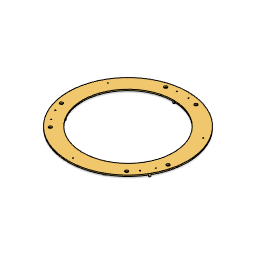
Hexapod Assembly (v6~recovered) (Autodesk Fusion 360 archive; units mm, degrees)
design "Bottom Plate"
Autodesk Fusion 360 part; units mm, degrees
sketch "Sketch1" plane through (0, 0, 0) normal (0, 1, 0) x (1, 0, 0)
  circle A0 centre (0, 0) radius 250
  circle A1 centre (0, 0) radius 230 construction
  circle A2 centre (63.3966, 221.0902) radius 6.5
  line L0 (63.3966, 221.0902) -> (0, 0) construction
  line L1 (0, 0) -> (0, 284.6738) construction
  line L2 (0, 0) -> (360.2208, 0) construction
  circle A3 centre (-63.3966, 221.0902) radius 6.5
  circle A4 centre (-223.168, -55.642) radius 6.5
  circle A5 centre (-159.7714, -165.4482) radius 6.5
  circle A6 centre (159.7714, -165.4482) radius 6.5
  circle A7 centre (223.168, -55.642) radius 6.5
  dimension "d13" = 500
  dimension "d14" = 460
  dimension "d15" = 13
  dimension "d60" = 16
  dimension "d62" = 360
  constraint coincident A0.centre A1.centre
  constraint concentric A0 A1
  constraint coincident A1 A2.centre
  constraint coincident A2.centre L0.start
  constraint vertical L1
  constraint perpendicular L1 L2
  constraint symmetric A2 L1 A3
  measures "d13" diameter of A0
  measures "d14" diameter of A1
  measures "d15" diameter of A2
  measures "d60" angle of L0 L1
extrude "Extrude8" add sketch "Sketch1" along normal blind 5
extrude "Extrude2" add sketch "Sketch1" along normal blind 5 contours A0 | A3 | A4 | A5 | A6 | A7
sketch "Sketch2" plane through (0, 0, 0) normal (0, -1, 0) x (1, 0, 0)
  circle A0 centre (63.3966, -221.0902) radius 6.5
  circle A1 centre (0, 0) radius 250
  circle A2 centre (0, 0) radius 230
  line L0 (0, 0) -> (-199.1858, -115) construction
  line L1 (0, 0) -> (0, -250) construction
  circle A3 centre (-199.1858, -115) radius 12.5
  circle A4 centre (199.1858, -115) radius 12.5
  circle A5 centre (0, 230) radius 12.5
  dimension "d21" = 460
  dimension "d22" = 60
  dimension "d23" = 25
  dimension "d25" = 360
  constraint coincident A1.centre A2.centre
  constraint coincident A2 L0.end
  constraint coincident A1 L1.end
  constraint vertical L1
  constraint coincident L0.end A3.centre
  measures "d21" diameter of A2
  measures "d22" angle of L0 L1
  measures "d23" diameter of A3
hole "Hole1" at (-199.1858, -7, -115) direction (0, 1, 0) diameter 4 depth 20 tip angle 180
pattern_circular "C-Pattern1" count 3 over 360 about axis through (0, 1.75, 0) along (0, 1, 0) of "Hole1"
sketch "Sketch3" plane through (0, 0, 0) normal (0, -1, 0) x (1, 0, 0)
  circle A0 centre (63.3966, -221.0902) radius 6.5
  circle A1 centre (0, 0) radius 250
  circle A2 centre (0, 0) radius 250
  circle A3 centre (0, 0) radius 12.5
  line L0 (-3, -12.1347) -> (-3, -249.982)
  line L1 (3, -12.1347) -> (3, -249.982)
  line L2 (12.0089, 3.4693) -> (217.9908, 122.3929)
  line L3 (9.0089, 8.6654) -> (214.9908, 127.5891)
  line L4 (-9.0089, 8.6654) -> (-214.9908, 127.5891)
  line L5 (-12.0089, 3.4693) -> (-217.9908, 122.3929)
  circle A4 centre (199.1858, -115) radius 2
  circle A5 centre (0, 230) radius 2
  circle A6 centre (-199.1858, -115) radius 2
  dimension "d34" = 500
  dimension "d42" = 25
  dimension "d45" = 6
  dimension "d48" = 360
  constraint concentric A1 A2
  constraint coincident A3 L0.start
  constraint coincident A1 L0.end
  constraint vertical L0
  constraint coincident A3 L1.start
  constraint coincident A1 L1.end
  constraint parallel L0 L1
  measures "d34" diameter of A2
  measures "d42" diameter of A3
  measures "d45" distance of L0 L1
extrude "Extrude5" add sketch "Sketch3" along normal blind 7 contours A1 A2 A3 L2 L3 | A1 A2 A3 L0 L1 | A3 | A1 A2 A3 L4 L5
fillet "Fillet1" radius 3 6 edges at (-9.0089, -3.5, 8.6654) (9.0089, -3.5, 8.6654) (-3, -3.5, -12.1347) (-12.0089, -3.5, 3.4693) (12.0089, -3.5, 3.4693) (3, -3.5, -12.1347)
sketch "Sketch4" plane through (0, 0, 0) normal (0, -1, 0) x (1, 0, 0)
  arc A0 (4.8387, -11.5255) -> (3, -14.2916) centre (6, -14.2916) ccw
  line L0 (3, -14.2916) -> (3, -249.982)
  arc A1 (3, -249.982) -> (217.9908, 122.3929) centre (0, 0) ccw
  line L1 (217.9908, 122.3929) -> (13.8769, 4.5477)
  arc A2 (13.8769, 4.5477) -> (12.4007, 1.5723) centre (15.3769, 1.9497) ccw
  arc A3 (4.8387, -11.5255) -> (12.4007, 1.5723) centre (0, 0) ccw
  circle A4 centre (63.3966, -221.0902) radius 6.5
  circle A5 centre (0, 0) radius 250 construction
  circle A6 centre (0, 0) radius 230 construction
  circle A7 centre (186.0739, 135.1906) radius 2
  line L2 (0, 0) -> (0, 80) construction
  line L3 (186.0739, 135.1906) -> (0, 0) construction
  line L4 (0, 0) -> (216.5064, 125) construction
  circle A8 centre (210.1155, 93.5494) radius 2
  circle A9 centre (-186.0739, 135.1906) radius 2
  circle A10 centre (-210.1155, 93.5494) radius 2
  circle A11 centre (-24.0415, -228.74) radius 2
  circle A12 centre (24.0415, -228.74) radius 2
  circle A13 centre (229.8599, -8.0269) radius 12.5
  line L5 (229.8599, -8.0269) -> (0, 0) construction
  line L6 (0, 0) -> (275.6577, -159.151) construction
  circle A14 centre (121.8814, -195.0511) radius 12.5
  circle A15 centre (-107.9785, 203.0779) radius 12.5
  circle A16 centre (107.9785, 203.0779) radius 12.5
  circle A17 centre (-121.8814, -195.0511) radius 12.5
  circle A18 centre (-229.8599, -8.0269) radius 12.5
  circle A19 centre (199.1858, -115) radius 2
  circle A20 centre (229.8599, -8.0269) radius 2
  circle A21 centre (121.8814, -195.0511) radius 2
  circle A22 centre (107.9785, 203.0779) radius 2
  circle A23 centre (-107.9785, 203.0779) radius 2
  circle A24 centre (-229.8599, -8.0269) radius 2
  circle A25 centre (-121.8814, -195.0511) radius 2
  dimension "d53" = 460
  dimension "d54" = 4
  dimension "d55" = 54
  dimension "d57" = 360
  dimension "d65" = 500
  dimension "d73" = 25
  dimension "d74" = 32
  dimension "d75" = 28
  dimension "d77" = 360
  dimension "d80" = 4
  dimension "d82" = 360
  constraint concentric A1 A5
  constraint concentric A5 A6
  constraint coincident A6 A7.centre
  constraint coincident A1.centre A3.centre
  constraint vertical L2
  constraint coincident A7.centre L3.start
  constraint coincident A5 L4.end
  constraint parallel L1 L4
  constraint symmetric A7 L4 A8
  constraint coincident A6 A13.centre
  constraint coincident A13.centre L5.start
  constraint symmetric A13 L6 A14
  constraint concentric A13 A20
  constraint symmetric L6 A20 A21
  measures "d53" diameter of A6
  measures "d54" diameter of A7
  measures "d55" angle of L2 L3
  measures "d65" diameter of A5
  measures "d73" diameter of A13
  measures "d74" angle of L1 L5
  measures "d75" angle of L5 L6
  measures "d80" diameter of A20
extrude "Extrude11" add sketch "Sketch4" along normal blind 7 contours A13 | A14 | A15 | A16 | A17 | A18
extrude "Extrude6" cut sketch "Sketch4" against normal blind 40 contours A7 | A8 | A9 | A10 | A11 | A12
extrude "Extrude9" cut sketch "Sketch1" along normal blind 35 contours A2 | A3 | A4 | A5 | A6 | A7
sketch "Sketch5" plane through (0, -7, 0) normal (0, -1, 0) x (1, 0, 0)
  line L0 (-3, -14.2916) -> (-3, -249.982)
  arc A0 (-3, -249.982) -> (3, -249.982) centre (0, 0) ccw
  line L1 (3, -249.982) -> (3, -14.2916)
  arc A1 (4.8387, -11.5255) -> (3, -14.2916) centre (6, -14.2916) ccw
  arc A2 (4.8387, -11.5255) -> (12.4007, 1.5723) centre (0, 0) ccw
  arc A3 (13.8769, 4.5477) -> (12.4007, 1.5723) centre (15.3769, 1.9497) ccw
  line L2 (13.8769, 4.5477) -> (217.9908, 122.3929)
  arc A4 (217.9908, 122.3929) -> (214.9908, 127.5891) centre (0, 0) ccw
  line L3 (214.9908, 127.5891) -> (10.8769, 9.7439)
  arc A5 (7.562, 9.9532) -> (10.8769, 9.7439) centre (9.3769, 12.342) ccw
  arc A6 (7.562, 9.9532) -> (-7.562, 9.9532) centre (0, 0) ccw
  arc A7 (-10.8769, 9.7439) -> (-7.562, 9.9532) centre (-9.3769, 12.342) ccw
  line L4 (-10.8769, 9.7439) -> (-214.9908, 127.5891)
  arc A8 (-214.9908, 127.5891) -> (-217.9908, 122.3929) centre (0, 0) ccw
  line L5 (-217.9908, 122.3929) -> (-13.8769, 4.5477)
  arc A9 (-12.4007, 1.5723) -> (-13.8769, 4.5477) centre (-15.3769, 1.9497) ccw
  arc A10 (-12.4007, 1.5723) -> (-4.8387, -11.5255) centre (0, 0) ccw
  arc A11 (-3, -14.2916) -> (-4.8387, -11.5255) centre (-6, -14.2916) ccw
  circle A12 centre (0, 0) radius 190
  dimension "d70" = 380
  constraint concentric A0 A12
  measures "d70" diameter of A12
extrude "Extrude10" cut sketch "Sketch5" against normal blind 50 contours L0 L1 A1 A2 A3 L2 L3 A5 A6 A7 L4 L5 A9 A10 A11 A12 | L0 L5 A9 A10 A11 A12 | L1 A1 A2 A3 L2 A12 | L3 A5 A6 A7 L4 A12
equation "hole_angle = 16 deg"
equation "hole_c_diameter = 460 mm"
equation "disk_diameter = 500 mm"
equation "hole_diameter = 13 mm"
equation "d13 = disk_diameter"
equation "d14 = hole_c_diameter"
equation "d15 = hole_diameter"
equation "d21 = hole_c_diameter"
equation "d60 = hole_angle"
equation "d70 = disk_diameter - 120 mm"

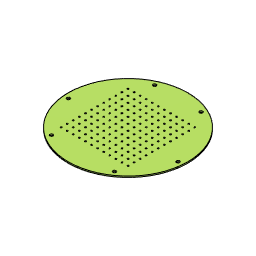
design "Top Plate"
Autodesk Fusion 360 part; units mm, degrees
sketch "Sketch2" plane through (0, 0, 0) normal (0, 1, 0) x (1, 0, 0)
  circle A0 centre (0, 0) radius 250
  circle A1 centre (0, 0) radius 230 construction
  line L0 (0, 0) -> (0, 300) construction
  circle A2 centre (97.2022, 208.4508) radius 6.5
  line L1 (97.2022, 208.4508) -> (0, 0) construction
  circle A3 centre (-97.2022, 208.4508) radius 6.5
  circle A4 centre (-229.1248, -20.0458) radius 6.5
  circle A5 centre (-131.9226, -188.405) radius 6.5
  circle A6 centre (131.9226, -188.405) radius 6.5
  circle A7 centre (229.1248, -20.0458) radius 6.5
  dimension "d52" = 500
  dimension "d53" = 460
  dimension "d54" = 13
  dimension "d55" = 25
  dimension "d57" = 360
  constraint coincident A0.centre A1.centre
  constraint vertical L0
  constraint coincident A1 A2.centre
  constraint coincident A2.centre L1.start
  constraint symmetric L0 A2 A3
  measures "d52" diameter of A0
  measures "d53" diameter of A1
  measures "d54" diameter of A2
  measures "d55" angle of L0 L1
extrude "Extrude4" add sketch "Sketch2" along normal blind 5
sketch "Sketch3" plane through (0, 5, 0) normal (0, 1, 0) x (-1, 0, 0)
  circle A0 centre (-97.2022, -208.4508) radius 6.5
  circle A1 centre (229.1248, 20.0458) radius 6.5
  circle A2 centre (97.2022, -208.4508) radius 6.5
  circle A3 centre (131.9226, 188.405) radius 6.5
  circle A4 centre (-131.9226, 188.405) radius 6.5
  circle A5 centre (-229.1248, 20.0458) radius 6.5
  circle A6 centre (0, 0) radius 250
  circle A7 centre (139.7, -139.7) radius 3
  line L0 (0, 0) -> (265, 0) construction
  line L1 (0, 0) -> (0, -270) construction
  circle A8 centre (114.3, -139.7) radius 3
  circle A9 centre (88.9, -139.7) radius 3
  circle A10 centre (63.5, -139.7) radius 3
  circle A11 centre (38.1, -139.7) radius 3
  circle A12 centre (12.7, -139.7) radius 3
  circle A13 centre (-12.7, -139.7) radius 3
  circle A14 centre (-38.1, -139.7) radius 3
  circle A15 centre (-63.5, -139.7) radius 3
  circle A16 centre (-88.9, -139.7) radius 3
  circle A17 centre (-114.3, -139.7) radius 3
  circle A18 centre (-139.7, -139.7) radius 3
  circle A19 centre (139.7, -114.3) radius 3
  circle A20 centre (114.3, -114.3) radius 3
  circle A21 centre (88.9, -114.3) radius 3
  circle A22 centre (63.5, -114.3) radius 3
  circle A23 centre (38.1, -114.3) radius 3
  circle A24 centre (12.7, -114.3) radius 3
  circle A25 centre (-12.7, -114.3) radius 3
  circle A26 centre (-38.1, -114.3) radius 3
  circle A27 centre (-63.5, -114.3) radius 3
  circle A28 centre (-88.9, -114.3) radius 3
  circle A29 centre (-114.3, -114.3) radius 3
  circle A30 centre (-139.7, -114.3) radius 3
  circle A31 centre (139.7, -88.9) radius 3
  circle A32 centre (114.3, -88.9) radius 3
  circle A33 centre (88.9, -88.9) radius 3
  circle A34 centre (63.5, -88.9) radius 3
  circle A35 centre (38.1, -88.9) radius 3
  circle A36 centre (12.7, -88.9) radius 3
  circle A37 centre (-12.7, -88.9) radius 3
  circle A38 centre (-38.1, -88.9) radius 3
  circle A39 centre (-63.5, -88.9) radius 3
  circle A40 centre (-88.9, -88.9) radius 3
  circle A41 centre (-114.3, -88.9) radius 3
  circle A42 centre (-139.7, -88.9) radius 3
  circle A43 centre (139.7, -63.5) radius 3
  circle A44 centre (114.3, -63.5) radius 3
  circle A45 centre (88.9, -63.5) radius 3
  circle A46 centre (63.5, -63.5) radius 3
  circle A47 centre (38.1, -63.5) radius 3
  circle A48 centre (12.7, -63.5) radius 3
  circle A49 centre (-12.7, -63.5) radius 3
  circle A50 centre (-38.1, -63.5) radius 3
  circle A51 centre (-63.5, -63.5) radius 3
  circle A52 centre (-88.9, -63.5) radius 3
  circle A53 centre (-114.3, -63.5) radius 3
  circle A54 centre (-139.7, -63.5) radius 3
  circle A55 centre (139.7, -38.1) radius 3
  circle A56 centre (114.3, -38.1) radius 3
  circle A57 centre (88.9, -38.1) radius 3
  circle A58 centre (63.5, -38.1) radius 3
  circle A59 centre (38.1, -38.1) radius 3
  circle A60 centre (12.7, -38.1) radius 3
  circle A61 centre (-12.7, -38.1) radius 3
  circle A62 centre (-38.1, -38.1) radius 3
  circle A63 centre (-63.5, -38.1) radius 3
  circle A64 centre (-88.9, -38.1) radius 3
  circle A65 centre (-114.3, -38.1) radius 3
  circle A66 centre (-139.7, -38.1) radius 3
  circle A67 centre (139.7, -12.7) radius 3
  circle A68 centre (114.3, -12.7) radius 3
  circle A69 centre (88.9, -12.7) radius 3
  circle A70 centre (63.5, -12.7) radius 3
  circle A71 centre (38.1, -12.7) radius 3
  circle A72 centre (12.7, -12.7) radius 3
  circle A73 centre (-12.7, -12.7) radius 3
  circle A74 centre (-38.1, -12.7) radius 3
  circle A75 centre (-63.5, -12.7) radius 3
  circle A76 centre (-88.9, -12.7) radius 3
  circle A77 centre (-114.3, -12.7) radius 3
  circle A78 centre (-139.7, -12.7) radius 3
  circle A79 centre (139.7, 12.7) radius 3
  circle A80 centre (114.3, 12.7) radius 3
  circle A81 centre (88.9, 12.7) radius 3
  circle A82 centre (63.5, 12.7) radius 3
  circle A83 centre (38.1, 12.7) radius 3
  circle A84 centre (12.7, 12.7) radius 3
  circle A85 centre (-12.7, 12.7) radius 3
  circle A86 centre (-38.1, 12.7) radius 3
  circle A87 centre (-63.5, 12.7) radius 3
  circle A88 centre (-88.9, 12.7) radius 3
  circle A89 centre (-114.3, 12.7) radius 3
  circle A90 centre (-139.7, 12.7) radius 3
  circle A91 centre (139.7, 38.1) radius 3
  circle A92 centre (114.3, 38.1) radius 3
  circle A93 centre (88.9, 38.1) radius 3
  circle A94 centre (63.5, 38.1) radius 3
  circle A95 centre (38.1, 38.1) radius 3
  circle A96 centre (12.7, 38.1) radius 3
  circle A97 centre (-12.7, 38.1) radius 3
  circle A98 centre (-38.1, 38.1) radius 3
  circle A99 centre (-63.5, 38.1) radius 3
  circle A100 centre (-88.9, 38.1) radius 3
  circle A101 centre (-114.3, 38.1) radius 3
  circle A102 centre (-139.7, 38.1) radius 3
  circle A103 centre (139.7, 63.5) radius 3
  circle A104 centre (114.3, 63.5) radius 3
  circle A105 centre (88.9, 63.5) radius 3
  circle A106 centre (63.5, 63.5) radius 3
  circle A107 centre (38.1, 63.5) radius 3
  circle A108 centre (12.7, 63.5) radius 3
  circle A109 centre (-12.7, 63.5) radius 3
  circle A110 centre (-38.1, 63.5) radius 3
  circle A111 centre (-63.5, 63.5) radius 3
  circle A112 centre (-88.9, 63.5) radius 3
  circle A113 centre (-114.3, 63.5) radius 3
  circle A114 centre (-139.7, 63.5) radius 3
  circle A115 centre (139.7, 88.9) radius 3
  circle A116 centre (114.3, 88.9) radius 3
  circle A117 centre (88.9, 88.9) radius 3
  circle A118 centre (63.5, 88.9) radius 3
  circle A119 centre (38.1, 88.9) radius 3
  circle A120 centre (12.7, 88.9) radius 3
  circle A121 centre (-12.7, 88.9) radius 3
  circle A122 centre (-38.1, 88.9) radius 3
  circle A123 centre (-63.5, 88.9) radius 3
  circle A124 centre (-88.9, 88.9) radius 3
  circle A125 centre (-114.3, 88.9) radius 3
  circle A126 centre (-139.7, 88.9) radius 3
  circle A127 centre (139.7, 114.3) radius 3
  circle A128 centre (114.3, 114.3) radius 3
  circle A129 centre (88.9, 114.3) radius 3
  circle A130 centre (63.5, 114.3) radius 3
  circle A131 centre (38.1, 114.3) radius 3
  circle A132 centre (12.7, 114.3) radius 3
  circle A133 centre (-12.7, 114.3) radius 3
  circle A134 centre (-38.1, 114.3) radius 3
  circle A135 centre (-63.5, 114.3) radius 3
  circle A136 centre (-88.9, 114.3) radius 3
  circle A137 centre (-114.3, 114.3) radius 3
  circle A138 centre (-139.7, 114.3) radius 3
  circle A139 centre (139.7, 139.7) radius 3
  circle A140 centre (114.3, 139.7) radius 3
  circle A141 centre (88.9, 139.7) radius 3
  circle A142 centre (63.5, 139.7) radius 3
  circle A143 centre (38.1, 139.7) radius 3
  circle A144 centre (12.7, 139.7) radius 3
  circle A145 centre (-12.7, 139.7) radius 3
  circle A146 centre (-38.1, 139.7) radius 3
  circle A147 centre (-63.5, 139.7) radius 3
  circle A148 centre (-88.9, 139.7) radius 3
  circle A149 centre (-114.3, 139.7) radius 3
  circle A150 centre (-139.7, 139.7) radius 3
  dimension "d60" = 6
  dimension "d61" = 139.7
  dimension "d62" = 139.7
  dimension "d65" = -279.4
  dimension "d66" = 0
  dimension "d69" = 0
  dimension "d70" = 279.4
  constraint coincident A6.centre L0.start
  constraint horizontal L0
  constraint perpendicular L0 L1
  measures "d60" diameter of A7
  measures "d61" distance of A7.centre L0
  measures "d62" distance of A7.centre L1
extrude "Extrude5" cut sketch "Sketch3" against normal blind 40 contours A7 | A8 | A9 | A10 | A11 | A12 | A13 | A14 | A15 | A16 | A17 | A18 | A19 | A20 | A21 | A22 | A23 | A24 | A25 | A26 | A27 | A28 | A29 | A30 | A31 | A32 | A33 | A34 | A35 | A36 | A37 | A38 | A39 | A40 | A41 | A42 | A43 | A44 | A45 | A46 | A47 | A48 | A49 | A50 | A51 | A52 | A53 | A54 | A55 | A56 | A57 | A58 | A59 | A60 | A61 | A62 | A63 | A64 | A65 | A66 | A67 | A68 | A69 | A70 | A71 | A72 | A73 | A74 | A75 | A76 | A77 | A78 | A79 | A80 | A81 | A82 | A83 | A84 | A85 | A86 | A87 | A88 | A89 | A90 | A91 | A92 | A93 | A94 | A95 | A96 | A97 | A98 | A99 | A100 | A101 | A102 | A103 | A104 | A105 | A106 | A107 | A108 | A109 | A110 | A111 | A112 | A113 | A114 | A115 | A116 | A117 | A118 | A119 | A120 | A121 | A122 | A123 | A124 | A125 | A126 | A127 | A128 | A129 | A130 | A131 | A132 | A133 | A134 | A135 | A136 | A137 | A138 | A139 | A140 | A141 | A142 | A143 | A144 | A145 | A146 | A147 | A148 | A149 | A150
equation "hole_angle = 25 deg"
equation "hole_c_diameter = 460 mm"
equation "hole_diameter = 13 mm"
equation "disk_diameter = 500 mm"
equation "disk_thickness = 5 mm"
equation "d13 = disk_diameter"
equation "d14 = hole_c_diameter"
equation "d15 = hole_diameter"
equation "d16 = hole_angle"
equation "d52 = disk_diameter"
equation "d53 = hole_c_diameter"
equation "d54 = hole_diameter"
equation "d55 = hole_angle"
equation "d61 = ( 279.4 / 2 ) * 1 mm"
